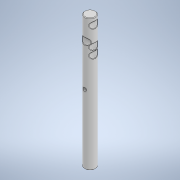
# Autodesk Inventor part: 80. Шток первой и второй передач
Saved by Autodesk Inventor 2021 (Build 250183000, 183)
## iProperties
Created: 2021-03-18
Part Number: 80. Шток первой и второй передач
Material: Типовые
Document SubType Name: Modeling
Designer: Данил
Density: 1 g/cm^3
Appearance: По умолчанию
Author: Данил
Autodesk Inventor part; units mm, degrees
ref_plane "YZ Plane" through (0, 0, 0) normal (1, 0, 0) x (0, 1, 0)
ref_plane "XZ Plane" through (0, 0, 0) normal (0, 1, 0) x (-1, 0, 0)
sketch "Эскиз1" plane through (0, 0, 0) normal (0, 0, 1) x (1, 0, 0)
  line L0 (0, 91.5) -> (0, -91.5)
  line L1 (0, -91.5) -> (6.75, -91.5)
  line L2 (7.5, -90.75) -> (7.5, 90.75)
  line L3 (6.75, 91.5) -> (0, 91.5)
  line L4 (7.5, -90.75) -> (6.75, -91.5)
  line L5 (7.5, 90.75) -> (6.75, 91.5)
  point P0 (0, 0)
  point P1 (0, 0)
  point P2 (7.5, -91.5)
  point P3 (7.5, 91.5)
  dimension "d0" = 183
  dimension "d1" = 15
  dimension "d2" = 0.75
  dimension "d3" = 45
  dimension "d4" = 0.75
  dimension "d5" = 45
  constraints: 12 end point, 4 point on line, 2 perpendicular, 1 coincident, 1 horizontal, 1 midpoint, 1 vertical
  measures "d0" distance of L0.start L0.end
  measures "d1" diameter of L2 L0
  measures "d2" distance of L2.start point (7.5, -91.5)
  measures "d3" angle of L2 L4
  measures "d4" distance of L2.end point (7.5, 91.5)
  measures "d5" angle of L2 L5
revolve "Вращение1" add sketch "Эскиз1" angle 360 about axis through (0, 91.5, 0) along (0, -1, 0)
sketch "Эскиз2" plane through (0, 0, 0) normal (0, 0, 1) x (1, 0, 0)
  arc A0 (7.5, 86.812772) -> (7.5, 78.187228) centre (9.1, 82.5) ccw
  line L0 (7.5, 90.75) -> (7.5, -90.75)
  line L1 (-7.5, 90.75) -> (-7.5, -90.75)
  line L2 (-6.75, 91.5) -> (6.75, 91.5)
  point P0 (0, 0)
  point P1 (4.5, 82.5)
  dimension "d7" = 12
  dimension "d8" = 4.6
  dimension "d9" = 9
  constraints: 3 point on circle, 2 point on line, 1 centre point, 1 horizontal alignment
  measures "d7" distance from line of L1 point (4.5, 82.5)
  measures "d8" radius of A0
  measures "d9" distance from line of L2 point (4.5, 82.5)
extrude "Выдавливание1" cut sketch "Эскиз2" against normal through all both and the other way through all
pattern_linear "Прямоуг.массив1" count 2 spacing 26 along (0, -1, 0) of "Выдавливание1"
pattern_linear "Прямоуг.массив2" count 2 spacing 10 along (0, -1, 0) of "Прямоуг.массив1"
ref_plane "РабПлоскость1" through (0, 0, -8) normal (0, 0, 1) x (1, 0, 0)
sketch "Эскиз3" plane through (0, 0, -8) normal (0, 0, 1) x (1, 0, 0)
  line L0 (0, 56.5) -> (0, -83.5) construction
  arc A0 (7.496925, 60.81163) -> (7.5, 52.187228) centre (9.1, 56.5) ccw
  point P0 (0, 0)
  dimension "d20" = 4.6
  dimension "d21" = 140
  constraints: 2 end point, 2 point on circle, 1 centre point, 1 coincident, 1 horizontal alignment, 1 vertical, 1 vertical alignment, 3 other
  measures "d20" radius of A0
  measures "d21" distance of L0.start L0.end
hole "Отверстие1" at (0, -83.5, -8) direction (0, 0, 1) diameter 4.5 depth 11 tip angle 120 countersink diameter 8.7 countersink angle 30
sketch "Эскиз4" plane through (0, 0, 0) normal (1, 0, 0) x (0, 1, 0)
  line L0 (-85.75, 3) -> (-83.5, 4.299038)
  line L1 (90.75, 7.5) -> (-90.75, 7.5)
  line L2 (90.75, -7.5) -> (-90.75, -7.5)
  arc A0 (58.050281, 7.5) -> (66.949719, 7.5) centre (62.5, 9.3) ccw
  point P0 (0, 0)
  point P1 (62.5, 4.5)
  dimension "d29" = 4.8
  dimension "d30" = 146
  dimension "d31" = 12
  constraints: 3 point on circle, 2 point on line, 1 centre point
  measures "d29" radius of A0
  measures "d30" distance of L0.end point (62.5, 4.5)
  measures "d31" distance from line of L2 point (62.5, 4.5)
extrude "Выдавливание2" cut sketch "Эскиз4" against normal through all both and the other way through all
fillet "Сопряжение2" radius 0.8 8 edges at (4.5, 82.4957, -6) (4.5, 82.4957, 6) (4.5, 56.4957, -6) (4.5, 56.4957, 6) (4.5, 46.4957, -6) (4.5, 46.4957, 6) (-6, 62.4998, 4.5) (6, 62.4993, 4.5)
sketch "Эскиз5" plane through (0, 0, 0) normal (0, 0, 1) x (1, 0, 0)
  line L0 (-6.75, 91.5) -> (6.75, 91.5) projected
  point P0 (0, 0)
  point P1 (0, 4.5)
  dimension "d37" = 87
  constraints: 1 vertical alignment
  measures "d37" distance from line of L0 point (0, 4.5)
hole "Отверстие2" at (0, 4.5, 0) direction (0, 0, -1) diameter 5 end through all both
equation "\"d4\" = d2"
equation "\"d5\" = d3"
